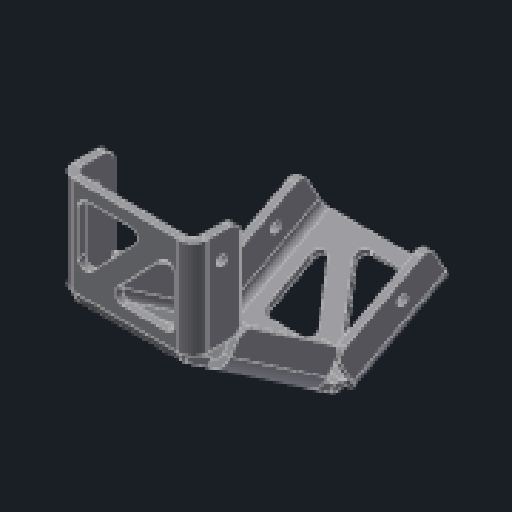
# Autodesk Inventor part: HipCoverTop
Saved by Autodesk Inventor 2025.2 (Build 292293000, 293)
## iProperties
Created: 2020-05-24
Part Number: HipCoverTop
Material: Generic
Document SubType Name: Sheet Metal
Designer: valer
Density: 1 g/cm^3
Sheet Metal Rule: Default
Appearance: Default
Author: valer
Autodesk Inventor part; units mm, degrees
ref_plane "YZ Plane" through (0, 0, 0) normal (1, 0, 0) x (0, 1, 0)
ref_plane "XZ Plane" through (0, 0, 0) normal (0, 1, 0) x (-1, 0, 0)
ref_plane "XY Plane" through (0, 0, 0) normal (0, 0, 1) x (1, 0, 0)
sketch "Base" plane through (0, 0, 0) normal (0, 0, 1) x (1, 0, 0)
  line L0 (0, 0) -> (44.58, 0)
  line L1 (44.58, 0) -> (44.58, -65.2018)
  line L2 (44.58, -65.2018) -> (0, -65.2018)
  line L3 (0, -65.2018) -> (0, 0)
  dimension "d0" = 65.2018
  dimension "d1" = 44.58
  measures "d0" distance of L2.end L0.start
  measures "d1" distance of L0.start L0.end
extrude "Plate1" add sketch "Base" along normal blind 4.7752
sketch "Sketch2" plane through (4.7752, 0, 4.7752) normal (-1, 0, 0) x (0, -1, 0)
  line L0 (65.2018, 0) -> (0, 0)
  line L1 (0, 0) -> (0, -31.75)
  line L2 (0, -31.75) -> (65.2018, -31.75)
  line L3 (65.2018, -31.75) -> (65.2018, 0)
  constraints: 6 end point, 1 horizontal, 1 perpendicular, 1 vertical
edge flange "MountFeature" height 31.75 angle 90 thickness 4.7752 bend radius 4.7752 thickness toward (-1, 0, 0) relief straight relief width 4.7752 relief depth 2.3876 edges at (0, -32.6009, 0) wall of the first edge with corners at (4.7752, -65.2018, 4.7752) (4.7752, 0, 4.7752) (4.7752, 0, -26.9748) (4.7752, -65.2018, -26.9748)
bend "Bend1"
corner "Corner1"
mirror "MirrorFeature" about plane through (44.58, 0, 0) normal (1, 0, 0)
sketch "GenerativeCut1" plane through (0, 0, 4.7752) normal (0, 0, 1) x (1, 0, 0)
  line L0 (12.7, -8.466667) -> (12.7, -56.735133)
  line L1 (12.7, -56.735133) -> (58.883171, -8.466667)
  line L2 (58.883171, -8.466667) -> (12.7, -8.466667)
  line L3 (79.6096, 0) -> (9.5504, 0)
  line L4 (30.276829, -56.735133) -> (76.46, -8.466667)
  line L5 (76.46, -8.466667) -> (76.46, -56.735133)
  line L6 (76.46, -56.735133) -> (30.276829, -56.735133)
  line L7 (58.883171, -8.466667) -> (76.46, -8.466667) construction
  line L8 (12.7, -56.735133) -> (30.276829, -56.735133) construction
  line L9 (0, -65.2018) -> (0, 0)
  line L10 (89.16, -65.2018) -> (89.16, 0)
  line L11 (79.6096, -65.2018) -> (9.5504, -65.2018)
  dimension "d23" = 8.46667
  dimension "d24" = 12.7
  dimension "d25" = 12.7
  dimension "d26" = 8.46667
  dimension "d27" = 12.7
  constraints: 16 end point, 2 parallel, 2 perpendicular, 1 collinear, 1 horizontal, 1 vertical
  measures "d23" distance between parallel lines of L3 L2
  measures "d24" distance between parallel lines of L9 L0
  measures "d25" distance between parallel lines of L5 L10
  measures "d26" distance between parallel lines of L11 L6
  measures "d27" distance between parallel lines of L4 L1
extrude "GenerativeCut1Feature" cut sketch "GenerativeCut1" against normal blind 25.4
fillet "GenerativeCut1FilletsFeature" radius 5.08 6 edges at (12.7, -8.4667, 2.3876) (12.7, -56.7351, 2.3876) (58.8832, -8.4667, 2.3876) (76.46, -8.4667, 2.3876) (30.2768, -56.7351, 2.3876) (76.46, -56.7351, 2.3876)
sketch "Sketch5" plane through (79.6096, -69.153616, -2.094587) normal (0, -0.8275708, 0.5613614) x (1, 0, 0)
  line L0 (-70.0592, 0) -> (0, 0)
  line L1 (0, 0) -> (0, 116.857987)
  line L2 (0, 116.857987) -> (-70.0592, 116.857987)
  line L3 (-70.0592, 116.857987) -> (-70.0592, 0)
  constraints: 6 end point, 1 horizontal, 1 perpendicular, 1 vertical
edge flange "KneeFlangeFeature" height 121.92 angle 55.85 thickness 4.7752 bend radius 4.7752 thickness toward (0, -0.8275708, 0.5613614) relief straight relief width 4.7752 relief depth 2.3876 edges at (44.58, -65.2018, 4.7752) wall of the first edge with corners at (9.5504, -69.153616, -2.094587) (79.6096, -69.153616, -2.094587) (79.6096, -134.753179, -98.802841) (9.5504, -134.753179, -98.802841)
bend "Bend2"
corner "Corner2"
sketch "Sketch6" plane through (9.5504, -135.016048, -103.728218) normal (0, -0.8826196, -0.4700879) x (1, 0, 0)
  line L0 (70.0592, 0) -> (0, 0)
  line L1 (0, 0) -> (0, -70.439967)
  line L2 (0, -70.439967) -> (70.0592, -70.439967)
  line L3 (70.0592, -70.439967) -> (70.0592, 0)
  constraints: 6 end point, 1 horizontal, 1 perpendicular, 1 vertical
edge flange "KneeBottomFlangeFeature" height 76.2 angle 62.19 thickness 4.7752 bend radius 4.7752 thickness toward (0, -0.8826196, -0.4700879) relief straight relief width 4.7752 relief depth 2.3876 edges at (44.58, -134.753179, -98.802841) wall of the first edge with corners at (79.6096, -135.016048, -103.728218) (9.5504, -135.016048, -103.728218) (9.5504, -101.903075, -165.899915) (79.6096, -101.903075, -165.899915)
bend "Bend3"
corner "Corner3"
sketch "Sketch8" plane through (4.7752, -130.801363, -101.483454) normal (-1, 0, 0) x (0, -1, 0)
  line L0 (-33.112974, -62.171697) -> (0, 0)
  line L1 (0, 0) -> (-19.593803, 10.435763)
  line L2 (-19.593803, 10.435763) -> (-52.706776, -51.735935)
  line L3 (-52.706776, -51.735935) -> (-33.112974, -62.171697)
  constraints: 6 end point, 1 perpendicular, 2 other
edge flange "KneeBottomSidesFeature" height 31.75 angle 90 thickness 4.7752 bend radius 4.7752 thickness toward (-1, 0, 0) relief straight relief width 4.7752 relief depth 2.3876 corner gap 4.7752 corner form 0 edges at (9.5504, -118.459562, -134.814066) (79.6096, -118.459562, -134.814066) wall of the first edge with corners at (4.7752, -97.68839, -163.655151) (4.7752, -130.801363, -101.483454) (4.7752, -111.20756, -91.047692) (4.7752, -78.094587, -153.219389)
bend "Bend4"
corner "Corner4"
fillet "OutsideFilletsFeature" radius 6.35 8 edges at (2.3876, -65.2018, -26.9748) (2.3876, 0, -26.9748) (2.3876, -111.2076, -91.0477) (86.7724, -78.0946, -153.2194) (2.3876, -78.0946, -153.2194) (86.7724, -111.2076, -91.0477) (86.7724, -65.2018, -26.9748) (86.7724, 0, -26.9748)
sketch "Sketch10" plane through (9.5504, -73.105432, 0.586026) normal (0, -0.8275708, 0.5613614) x (1, 0, 0)
  line L0 (-4.7752, -15.902021) -> (-9.5504, -15.902021)
  line L1 (-4.7752, -99.451558) -> (-9.5504, -99.451558)
  line L2 (-9.5504, -18.442021) -> (0, -18.442021)
  line L3 (0, -18.442021) -> (0, -96.911558)
  line L4 (0, -96.911558) -> (-9.5504, -96.911558)
  line L5 (-9.5504, -96.911558) -> (-9.5504, -18.442021)
  line L6 (-9.5504, 0) -> (-9.5504, -13.116666)
  line L7 (0, 0) -> (0, -116.857987)
  point P0 (-9.5504, 40.55359)
  dimension "d65" = 2.54
  dimension "d66" = 2.54
  constraints: 8 end point, 2 collinear, 2 parallel, 1 horizontal, 1 perpendicular
  measures "d65" distance between parallel lines of L0 L2
  measures "d66" distance between parallel lines of L1 L4
sheet face with bend "SideFlangeBaseFeature" sketch "Sketch10" thickness 4.7752 toward (0, 0.8275708, -0.5613614) bend radius 4.7752 relief straight relief width 4.7752 relief depth 2.3876
bend "Bend5"
sketch "Sketch11" plane through (4.7752, -83.45807, -14.676051) normal (-1, 0, 0) x (0, -1, 0)
  line L0 (44.049769, -64.939095) -> (0, 0)
  line L1 (0, 0) -> (-21.020298, -14.25858)
  line L2 (-21.020298, -14.25858) -> (23.029472, -79.197675)
  line L3 (23.029472, -79.197675) -> (44.049769, -64.939095)
  constraints: 6 end point, 1 perpendicular, 2 other
edge flange "SideFlangeFeature" height 25.4 angle 90 thickness 4.7752 bend radius 4.7752 thickness toward (-1, 0, 0) relief straight relief width 4.7752 relief depth 2.3876 edges at (0, -101.531139, -49.826212) wall of the first edge with corners at (4.7752, -127.50784, -79.615147) (4.7752, -83.45807, -14.676051) (4.7752, -62.437773, -28.934631) (4.7752, -106.487542, -93.873726)
bend "Bend6"
corner "Corner5"
ref_plane "MiddlePlane" through (44.58, -97.68839, -163.655151) normal (-1, 0, 0) x (0, -0.4700879, 0.8826196)
mirror "SideFlangeMirrorFeature" about plane through (44.58, -97.68839, -163.655151) normal (-1, 0, 0) of "SideFlangeFeature"
fillet "SideFlangeFilletsFeature" radius 6.35 4 edges at (2.3876, -106.4875, -93.8737) (86.7724, -106.4875, -93.8737) (2.3876, -62.4378, -28.9346) (86.7724, -62.4378, -28.9346)
sketch "Rais" plane through (9.5504, -73.105432, 0.586026) normal (0, -0.8275708, 0.5613614) x (1, 0, 0)
  line L0 (70.0592, 0) -> (0, 0) construction
  line L1 (0, -116.857987) -> (70.0592, -116.857987) construction
  line L2 (0, 0) -> (70.0592, 0) construction
  line L3 (35.0296, 0) -> (35.0296, -116.857987) construction
  line L4 (0, -116.857987) -> (70.0592, -116.857987) construction
  line L5 (26.819728, -42.590128) -> (17.839472, -33.609872) construction
  line L6 (24.574664, -44.835192) -> (15.594408, -35.854936)
  line L7 (20.084536, -31.364808) -> (29.064792, -40.345064)
  arc A0 (24.574664, -44.835192) -> (29.064792, -40.345064) centre (26.819728, -42.590128) ccw
  arc A1 (20.084536, -31.364808) -> (15.594408, -35.854936) centre (17.839472, -33.609872) ccw
  line L8 (0, -18.442021) -> (0, -96.911558) construction
  line L9 (0, -57.676789) -> (70.0592, -57.676789) construction
  line L10 (70.0592, -96.911558) -> (70.0592, -18.442021) construction
  line L11 (45.484536, -44.835192) -> (54.464792, -35.854936)
  line L12 (49.974664, -31.364808) -> (40.994408, -40.345064)
  arc A2 (40.994408, -40.345064) -> (45.484536, -44.835192) centre (43.239472, -42.590128) ccw
  arc A3 (54.464792, -35.854936) -> (49.974664, -31.364808) centre (52.219728, -33.609872) ccw
  line L13 (24.574664, -70.518387) -> (15.594408, -79.498643)
  line L14 (20.084536, -83.988771) -> (29.064792, -75.008515)
  arc A4 (29.064792, -75.008515) -> (24.574664, -70.518387) centre (26.819728, -72.763451) ccw
  arc A5 (15.594408, -79.498643) -> (20.084536, -83.988771) centre (17.839472, -81.743707) ccw
  line L15 (45.484536, -70.518387) -> (54.464792, -79.498643)
  arc A6 (49.974664, -83.988771) -> (54.464792, -79.498643) centre (52.219728, -81.743707) ccw
  line L16 (49.974664, -83.988771) -> (40.994408, -75.008515)
  arc A7 (45.484536, -70.518387) -> (40.994408, -75.008515) centre (43.239472, -72.763451) ccw
  point P0 (-9.5504, 40.55359)
  point P1 (22.3296, -38.1)
  dimension "d101" = 3.175
  dimension "d102" = 12.7
  dimension "d103" = 12.7
  dimension "d104" = 38.1
  dimension "d105" = 45
  constraints: 24 end point, 18 symmetric about line, 16 point on circle, 8 centre point, 5 midpoint, 4 tangent, 1 parallel, 6 other
  measures "d101" radius of A1
  measures "d102" distance from line of L3 point (22.33, -38.1)
  measures "d103" distance of L5.start L5.end
  measures "d104" distance from line of L0 point (22.33, -38.1)
  measures "d105" angle of L3 L5
extrude "RailsFeature" cut sketch "Rais" against normal blind 25.4
sketch "GenerativeCut2" plane through (9.5504, -139.230734, -105.972981) normal (0, -0.8826196, -0.4700879) x (1, 0, 0)
  line L0 (8.466667, -8.466667) -> (8.466667, -61.9733)
  line L1 (8.466667, -61.9733) -> (46.069949, -8.466667)
  line L2 (46.069949, -8.466667) -> (8.466667, -8.466667)
  line L3 (23.989251, -61.9733) -> (61.592533, -8.466667)
  line L4 (61.592533, -8.466667) -> (61.592533, -61.9733)
  line L5 (61.592533, -61.9733) -> (23.989251, -61.9733)
  line L6 (46.069949, -8.466667) -> (61.592533, -8.466667) construction
  line L7 (8.466667, -61.9733) -> (23.989251, -61.9733) construction
  line L8 (70.0592, 0) -> (0, 0)
  line L9 (0, -70.439967) -> (0, 0)
  line L10 (70.0592, -70.439967) -> (0, -70.439967)
  line L11 (70.0592, 0) -> (70.0592, -70.439967)
  point P0 (-9.5504, 28.083155)
  dimension "d124" = 12.7
  dimension "d125" = 8.46667
  dimension "d126" = 8.46667
  dimension "d127" = 8.46667
  dimension "d128" = 8.46667
  constraints: 16 end point, 2 perpendicular, 1 collinear, 1 horizontal, 1 parallel, 1 vertical
  measures "d124" distance between parallel lines of L3 L1
  measures "d125" distance between parallel lines of L8 L2
  measures "d126" distance between parallel lines of L9 L0
  measures "d127" distance between parallel lines of L11 L4
  measures "d128" distance between parallel lines of L10 L5
extrude "GenerativeCut2Feature" cut sketch "GenerativeCut2" against normal blind 25.4 contours L2 L1 L0 | L3 L4 L5
fillet "GenerativeCut2FilletsFeature" radius 5.08 6 edges at (18.0171, -133.1433, -112.3234) (55.6203, -133.1433, -112.3234) (18.0171, -107.9905, -159.5495) (33.5397, -107.9905, -159.5495) (71.1429, -133.1433, -112.3234) (71.1429, -107.9905, -159.5495)
sketch "Sketch17" plane through (0, -97.68839, -163.655151) normal (-1, 0, 0) x (0, -0.4700879, 0.8826196)
  line L0 (90.80282, 141.860385) -> (91.83694, 154.518213) construction
  arc A0 (90.80282, 141.860385) -> (97.131734, 141.343325) centre (93.967277, 141.601855) ccw construction
  line L1 (98.165854, 154.001153) -> (97.131734, 141.343325) construction
  arc A1 (98.165854, 154.001153) -> (91.83694, 154.518213) centre (95.001397, 154.259683) ccw construction
  line L2 (106.832455, 106.768684) -> (119.516068, 107.41362) construction
  arc A2 (106.832455, 106.768684) -> (107.154923, 100.426877) centre (106.993689, 103.59778) ccw construction
  line L3 (119.838537, 101.071813) -> (107.154923, 100.426877) construction
  arc A3 (119.838537, 101.071813) -> (119.516068, 107.41362) centre (119.677302, 104.242717) ccw construction
  arc A4 (68.314863, 17.539961) -> (62.3, 15.504298) centre (65.307431, 16.52213) ccw construction
  line L4 (66.371326, 3.474572) -> (62.3, 15.504298) construction
  arc A5 (66.371326, 3.474572) -> (72.386189, 5.510235) centre (69.378758, 4.492404) ccw construction
  line L5 (68.314863, 17.539961) -> (72.386189, 5.510235) construction
  line L6 (22.609123, 5.807043) -> (24.669095, 18.338863) construction
  arc A6 (30.935005, 17.308877) -> (24.669095, 18.338863) centre (27.80205, 17.82387) ccw construction
  line L7 (30.935005, 17.308877) -> (28.875033, 4.777057) construction
  arc A7 (22.609123, 5.807043) -> (28.875033, 4.777057) centre (25.742078, 5.29205) ccw construction
  circle A8 centre (93.967277, 141.601855) radius 3.175
  line L8 (27.80205, 17.82387) -> (25.742078, 5.29205) construction
  circle A9 centre (26.772064, 11.55796) radius 3.175
  line L9 (119.677302, 104.242717) -> (106.993689, 103.59778) construction
  line L10 (65.307431, 16.52213) -> (69.378758, 4.492404) construction
  point P0 (98.523122, 163.15399)
  constraints: 6 end point, 1 centre point, 1 coincident, 1 midpoint, 1 tangent, 3 other
extrude "Cut1" cut sketch "Sketch17" against normal through all
equation "\"d25\" = d24"
equation "\"d26\" = d23"
equation "\"d27\" = d24"
equation "\"d124\" = d121"
equation "\"d132\" = Thickness"
equation "\"d2\" = Thickness"
equation "\"d3\" = BendReliefWidth"
equation "\"d4\" = BendReliefDepth"
equation "\"d5\" = MinimumRemnant"
equation "\"d6\" = TransitionRadius"
equation "\"d9\" = BendRadius"
equation "\"d10\" = CornerReliefSize"
equation "\"d11\" = GapSize"
equation "\"d12\" = JacobiRadiusSize"
equation "\"d31\" = BendReliefWidth"
equation "\"d32\" = BendReliefDepth"
equation "\"d33\" = MinimumRemnant"
equation "\"d34\" = TransitionRadius"
equation "\"d37\" = BendRadius"
equation "\"d38\" = CornerReliefSize"
equation "\"d39\" = GapSize"
equation "\"d40\" = JacobiRadiusSize"
equation "\"d41\" = BendReliefWidth"
equation "\"d42\" = BendReliefDepth"
equation "\"d43\" = MinimumRemnant"
equation "\"d44\" = TransitionRadius"
equation "\"d47\" = BendRadius"
equation "\"d48\" = CornerReliefSize"
equation "\"d49\" = GapSize"
equation "\"d50\" = JacobiRadiusSize"
equation "\"d51\" = BendReliefWidth"
equation "\"d52\" = BendReliefDepth"
equation "\"d53\" = MinimumRemnant"
equation "\"d54\" = TransitionRadius"
equation "\"d57\" = BendRadius"
equation "\"d58\" = CornerReliefSize"
equation "\"d59\" = GapSize"
equation "\"d60\" = JacobiRadiusSize"
equation "\"d66\" = d65"
equation "\"d67\" = BendRadius"
equation "\"d68\" = BendReliefWidth"
equation "\"d70\" = MinimumRemnant"
equation "\"d69\" = BendReliefDepth"
equation "\"d71\" = TransitionRadius"
equation "\"d72\" = BendReliefWidth"
equation "\"d73\" = BendReliefDepth"
equation "\"d74\" = MinimumRemnant"
equation "\"d75\" = TransitionRadius"
equation "\"d78\" = BendRadius"
equation "\"d79\" = CornerReliefSize"
equation "\"d80\" = GapSize"
equation "\"d81\" = JacobiRadiusSize"
equation "\"BendRadius\" = Thickness"
equation "\"BendReliefWidth\" = Thickness"
equation "\"BendReliefDepth\" = 0.5 * Thickness"
equation "\"CornerReliefSize\" = 4 * Thickness"
equation "\"MinimumRemnant\" = 2 * Thickness"
equation "\"TransitionRadius\" = BendRadius"
equation "\"JacobiRadiusSize\" = BendRadius"
equation "\"GapSize\" = Thickness"
equation "\"d121\" = 12.7"
equation "\"Thickness\" = 4.7752"
body "Solid1"
